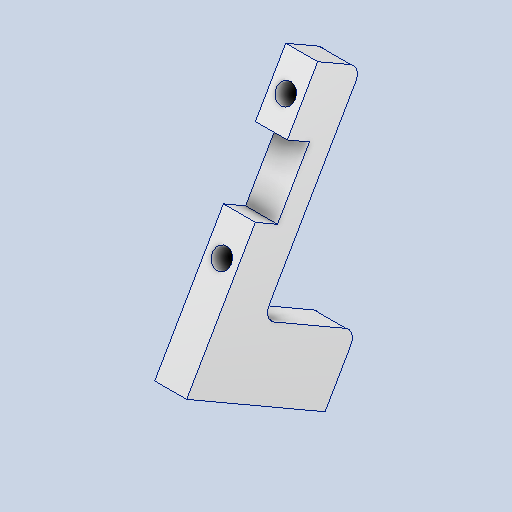
# Autodesk Inventor part: belt_liner_v2_Plate_5
Saved by Autodesk Inventor 2025.2 (Build 292293000, 293)
## iProperties
Created: 2025-01-06
Part Number: belt_liner_v2_Plate_5
Material: アルミニウム 6061
Document SubType Name: Modeling
Designer: haruy
Density: 2.7 g/cm^3
Appearance: アルミニウム - フラット
Author: haruy
Autodesk Inventor part; units mm, degrees
ref_plane "YZ Plane" through (0, 0, 0) normal (1, 0, 0) x (0, 1, 0)
ref_plane "XZ Plane" through (0, 0, 0) normal (0, 1, 0) x (-1, 0, 0)
ref_plane "XY Plane" through (0, 0, 0) normal (0, 0, 1) x (1, 0, 0)
derived "belt_liner_v2_Sketch_Base.ipt"
sketch "スケッチ1" plane through (300, 0, 0) normal (1, 0, 0) x (0, 1, 0)
  circle A0 centre (0, 0) radius 22.36
  circle A1 centre (742.4003, -428.625) radius 23.875 construction
  line L0 (0, 0) -> (0, -985.832)
  line L1 (4.6934, 56.2493) -> (12.1934, 69.2396)
  line L2 (12.1934, 69.2396) -> (479.8471, -200.7604)
  line L3 (479.8471, -200.7604) -> (472.3471, -213.7507)
  line L4 (472.3471, -213.7507) -> (4.6934, 56.2493)
  line L5 (0, 0) -> (742.4003, -428.625)
  line L6 (-43.5991, -27.3958) -> (-51.0991, -40.3862)
  line L7 (-51.0991, -40.3862) -> (711.0033, -480.3862)
  line L8 (711.0033, -480.3862) -> (718.5033, -467.3958)
  line L9 (718.5033, -467.3958) -> (-43.5991, -27.3958)
  line L10 (-64.8558, 113.724) -> (-64.8558, 113.724)
  line L11 (4.6934, 56.2493) -> (0.3513, 58.7562)
  line L12 (0.3513, 58.7562) -> (-2.1487, 54.426)
  line L13 (-2.1487, 54.426) -> (2.1934, 51.9191)
  line L14 (2.1934, 51.9191) -> (4.6934, 56.2493)
  line L15 (472.3471, -213.7507) -> (374.1722, -157.0694)
  line L16 (0, -985.832) -> (0, 0)
  circle A2 centre (0, 0) radius 12.5
  circle A3 centre (0, 0) radius 15
  line L17 (0, 0) -> (0, 0)
  circle A4 centre (0, 0) radius 24.06 construction
  line L18 (0, 0) -> (0, 0)
  line L19 (0, 0) -> (0, 0)
  line L20 (-43.5991, -27.3958) -> (-41.0991, -23.0657)
  line L21 (-41.0991, -23.0657) -> (28.9181, -63.4901)
  line L22 (32.4803, -71.3202) -> (-43.5991, -27.3958)
  line L23 (85.8056, 26.7396) -> (479.8471, -200.7604)
  line L24 (479.8471, -200.7604) -> (482.5971, -195.9972)
  circle A5 centre (742.4003, -428.625) radius 5
  line L25 (718.5033, -467.3958) -> (692.5225, -452.3958)
  line L26 (692.5225, -452.3958) -> (695.0225, -448.0657)
  line L27 (695.0225, -448.0657) -> (721.0033, -463.0657)
  line L28 (721.0033, -463.0657) -> (718.5033, -467.3958)
  circle A6 centre (738.0702, -426.125) radius 5.1
  line L29 (742.4003, -428.625) -> (511.0389, -295.0485)
  circle A7 centre (759.7208, -438.625) radius 5.1
  line L30 (740.6202, -421.7083) -> (762.2708, -434.2083)
  line L31 (735.5202, -430.5417) -> (757.1708, -443.0417)
  circle A8 centre (742.4003, -428.625) radius 22.175 construction
  line L32 (792.3761, -398.5196) -> (776.3761, -426.2324)
  line L33 (776.3761, -426.2324) -> (785.0364, -431.2324)
  line L34 (785.0364, -431.2324) -> (801.0364, -403.5196)
  line L35 (801.0364, -403.5196) -> (792.3761, -398.5196)
  circle A9 centre (738.0702, -426.125) radius 10.1 construction
  circle A10 centre (759.7208, -438.625) radius 10.1 construction
  line L36 (743.1202, -417.3781) -> (764.7708, -429.8781) construction
  line L37 (733.0202, -434.8719) -> (754.6708, -447.3719) construction
  line L38 (743.1202, -417.3781) -> (732.6663, -411.3426) construction
  line L39 (729.3233, -421.075) -> (734.3733, -412.3281) construction
  line L40 (764.7708, -429.8781) -> (773.0938, -434.6834) construction
  line L41 (773.0938, -434.6834) -> (773.431, -434.8781)
  line L42 (0.3513, 58.7562) -> (-2.1487, 54.426)
  line L43 (-2.1487, 54.426) -> (100.4873, -4.8309)
  line L44 (100.4873, -4.8309) -> (102.9873, -0.5007)
  line L45 (102.9873, -0.5007) -> (0.3513, 58.7562)
  line L46 (-51.0991, -40.3862) -> (-51.0991, -619.9209)
  line L47 (754.6708, -447.3719) -> (764.7708, -429.8781)
  line L48 (764.7708, -429.8781) -> (773.431, -434.8781)
  line L49 (773.431, -434.8781) -> (763.331, -452.3719)
  line L50 (763.331, -452.3719) -> (754.6708, -447.3719) construction
  line L51 (479.8471, -200.7604) -> (472.3471, -213.7507)
  line L52 (472.3471, -213.7507) -> (896.6996, -458.7507)
  line L53 (896.6996, -458.7507) -> (904.1996, -445.7603)
  line L54 (904.1996, -445.7603) -> (479.8471, -200.7604)
  line L55 (-12.1522, -2.9282) -> (-38.1087, -47.8862)
  line L56 (-12.1522, -2.9282) -> (25.1838, 61.7396)
  circle A11 centre (38.0844, 34.0842) radius 1.5
  circle A12 centre (59.7351, 21.5842) radius 1.5
  circle A13 centre (711.093, -460.2307) radius 1.5
  circle A14 centre (0, 0) radius 60
  line L57 (54.6948, -84.1458) -> (57.1948, -79.8157)
  line L58 (100.4873, -4.8309) -> (57.1948, -79.8157)
  circle A15 centre (81.3857, 9.0842) radius 1.5
  circle A16 centre (742.4003, -428.625) radius 6 construction
  circle A17 centre (0, 0) radius 24.06 construction
  circle A18 centre (0, 0) radius 24.06
  circle A19 centre (742.4003, -428.625) radius 24.06
  line L59 (754.4303, -407.7884) -> (12.03, 20.8366)
  circle A20 centre (725.8592, -419.075) radius 4
  circle A21 centre (725.8592, -419.075) radius 1.5
  circle A22 centre (742.4003, -428.625) radius 18.525 construction
  circle A23 centre (748.9869, -417.4167) radius 4
  line L60 (737.4369, -437.4219) -> (742.4869, -428.675)
  circle A24 centre (748.9869, -417.4167) radius 1.5
  line L61 (734.3733, -412.3281) -> (737.8233, -406.3526) construction
  line L62 (737.8233, -406.3526) -> (776.881, -428.9026)
  line L63 (773.431, -434.8781) -> (776.881, -428.9026)
  line L64 (737.8233, -406.3526) -> (723.6503, -415.7402)
  line L65 (720.8233, -435.7974) -> (759.881, -458.3474)
  line L66 (720.8233, -435.7974) -> (721.8667, -418.8295)
  line L67 (763.331, -452.3719) -> (759.881, -458.3474)
  circle A25 centre (735.9869, -439.9333) radius 4
  circle A26 centre (735.9869, -439.9333) radius 1.5
  circle A27 centre (300.5299, 58.6531) radius 120
  line L68 (24.7883, 15.78) -> (16.128, 20.78) construction
  line L69 (896.6996, -458.7507) -> (870.7188, -443.7507)
  line L70 (870.7188, -443.7507) -> (868.2188, -448.0808)
  line L71 (868.2188, -448.0808) -> (894.1996, -463.0808)
  line L72 (894.1996, -463.0808) -> (896.6996, -458.7507)
  circle A28 centre (886.7893, -455.9158) radius 1.5
  line L73 (100.4873, -4.8309) -> (102.9873, -0.5007)
  line L74 (102.9873, -0.5007) -> (112.9466, -6.2507)
  line L75 (112.9466, -6.2507) -> (110.4466, -10.5809)
  line L76 (110.4466, -10.5809) -> (100.4873, -4.8309)
  circle A29 centre (878.129, -450.9158) radius 1.5
  circle A30 centre (702.4328, -455.2307) radius 1.5
  line L77 (28.9181, -63.4901) -> (57.1948, -79.8157)
  line L78 (479.8471, -200.7604) -> (482.5971, -195.9972)
  line L79 (121.4466, 8.4717) -> (179.9033, -25.2783)
  line L80 (179.9033, -25.2783) -> (182.4033, -20.9482)
  line L81 (182.4033, -20.9482) -> (123.9466, 12.8018)
  line L82 (123.9466, 12.8018) -> (121.4466, 8.4717)
  circle A31 centre (135.9059, 10.5159) radius 4
  circle A32 centre (135.9059, 10.5159) radius 11
  circle A33 centre (161.8867, -4.4841) radius 4
  circle A34 centre (161.8867, -4.4841) radius 11
  line L83 (131.87, -4.4745) -> (128.37, -10.5366)
  line L84 (128.37, -10.5366) -> (147.4226, -21.5366)
  line L85 (147.4226, -21.5366) -> (150.9226, -15.4745)
  line L86 (150.9226, -15.4745) -> (131.87, -4.4745)
  line L87 (141.3963, -9.9745) -> (137.8963, -16.0366)
  line L88 (157.8508, -19.4745) -> (154.3508, -25.5366)
  line L89 (154.3508, -25.5366) -> (173.4033, -36.5366)
  line L90 (173.4033, -36.5366) -> (176.9033, -30.4745)
  line L91 (176.9033, -30.4745) -> (157.8508, -19.4745)
  line L92 (167.377, -24.9745) -> (163.877, -31.0366)
  line L93 (8.4434, 62.7444) -> (900.4496, -452.2555)
  line L94 (170.4033, -41.7328) -> (167.9033, -46.0629)
  line L95 (111.9466, -7.9828) -> (170.4033, -41.7328)
  line L96 (167.9033, -46.0629) -> (109.4466, -12.3129)
  line L97 (109.4466, -12.3129) -> (111.9466, -7.9828)
  circle A35 centre (117.4059, -21.527) radius 11
  circle A36 centre (117.4059, -21.527) radius 4
  circle A37 centre (143.3867, -36.527) radius 11
  circle A38 centre (143.3867, -36.527) radius 4
  line L98 (140.9322, -2.7783) -> (147.8604, -6.7783)
  line L99 (147.8604, -6.7783) -> (138.3604, -23.2328)
  line L100 (138.3604, -23.2328) -> (131.4322, -19.2328)
  line L101 (131.4322, -19.2328) -> (140.9322, -2.7783)
  line L102 (166.9129, -17.7783) -> (173.8411, -21.7783)
  line L103 (173.8411, -21.7783) -> (164.3411, -38.2328)
  line L104 (164.3411, -38.2328) -> (157.4129, -34.2328)
  line L105 (157.4129, -34.2328) -> (166.9129, -17.7783)
  line L106 (109.4466, -12.3129) -> (96.9466, -33.9636)
  line L107 (96.9466, -33.9636) -> (105.6069, -38.9636)
  line L108 (105.6069, -38.9636) -> (118.1069, -17.3129)
  line L109 (118.1069, -17.3129) -> (109.4466, -12.3129)
  line L110 (109.4466, -12.3129) -> (144.9536, -32.8129)
  line L111 (144.9536, -32.8129) -> (140.9536, -39.7411)
  line L112 (140.9536, -39.7411) -> (105.4466, -19.2411)
  line L113 (105.4466, -19.2411) -> (109.4466, -12.3129)
  line L114 (128.9322, -23.5629) -> (135.8604, -27.5629)
  line L115 (135.8604, -27.5629) -> (134.3604, -30.161)
  line L116 (134.3604, -30.161) -> (127.4322, -26.161)
  line L117 (127.4322, -26.161) -> (128.9322, -23.5629)
  circle A39 centre (-7.7081, -45.2307) radius 1.25
  circle A40 centre (13.9426, -57.7307) radius 1.25
  circle A41 centre (35.5932, -70.2307) radius 1.25
  circle A42 centre (300.5299, 58.6531) radius 130
  line L118 (300.5299, 58.6531) -> (196.6069, 118.6531)
  line L119 (300.5299, 58.6531) -> (184.6188, 27.5948)
  line L120 (300.5299, 58.6531) -> (269.4716, 174.5642)
  line L121 (272.4716, 179.7603) -> (181.6188, 22.3986)
  line L122 (181.6188, 22.3986) -> (176.4227, 25.3986)
  line L123 (176.4227, 25.3986) -> (267.2755, 182.7603)
  line L124 (267.2755, 182.7603) -> (272.4716, 179.7603)
  line L125 (300.5299, 58.6531) -> (235.5299, -53.9302)
  line L126 (791.3761, -400.2516) -> (788.8761, -404.5817)
  line L127 (788.8761, -404.5817) -> (847.3329, -438.3317)
  line L128 (847.3329, -438.3317) -> (849.8329, -434.0016)
  line L129 (849.8329, -434.0016) -> (791.3761, -400.2516)
  line L130 (849.8329, -434.0016) -> (847.3329, -438.3317)
  line L131 (847.3329, -438.3317) -> (867.2188, -449.8129)
  line L132 (867.2188, -449.8129) -> (869.7188, -445.4828)
  line L133 (869.7188, -445.4828) -> (849.8329, -434.0016)
  line L134 (737.8233, -406.3526) -> (868.2188, -448.0808)
  circle A43 centre (742.4003, -428.625) radius 34.06
  line L135 (859.2446, -445.209) -> (862.7446, -439.1468)
  circle A44 centre (742.4869, -428.675) radius 8.5
  line L136 (126.0662, -26.527) -> (134.7264, -31.527)
  line L137 (134.7264, -31.527) -> (137.2264, -27.1969)
  line L138 (137.2264, -27.1969) -> (128.5662, -22.1969)
  line L139 (128.5662, -22.1969) -> (126.0662, -26.527)
  line L140 (253.2022, 236.6791) -> (109.4466, -12.3129)
  line L141 (249.3989, -49.9085) -> (244.3828, -58.5967)
  line L142 (244.3828, -58.5967) -> (167.9033, -46.0629)
  line L143 (181.6188, 22.3986) -> (198.8709, -5.1077)
  line L144 (267.2755, 182.7603) -> (268.3404, 184.6048)
  circle A45 centre (127.0267, 8.1368) radius 1.5
  circle A46 centre (176.8232, -20.6132) radius 1.5
  circle A47 centre (115.0267, -12.6479) radius 1.5
  circle A48 centre (164.8232, -41.3979) radius 1.5
  line L145 (176.4227, 25.3986) -> (179.4227, 30.5948)
  line L146 (179.4227, 30.5948) -> (175.0925, 33.0948)
  line L147 (175.0925, 33.0948) -> (172.0925, 27.8986)
  line L148 (172.0925, 27.8986) -> (176.4227, 25.3986)
  line L149 (267.2755, 182.7603) -> (264.2755, 177.5642)
  line L150 (264.2755, 177.5642) -> (259.9453, 180.0642)
  line L151 (259.9453, 180.0642) -> (262.9453, 185.2603)
  line L152 (262.9453, 185.2603) -> (267.2755, 182.7603)
  circle A49 centre (263.6104, 181.4122) radius 1.5
  line L153 (268.3404, 184.6048) -> (262.9453, 185.2603)
  line L154 (262.9453, 185.2603) -> (242.1446, 174.8045)
  circle A50 centre (175.7576, 29.2467) radius 1.5
  line L155 (894.1996, -463.0808) -> (718.5033, -467.3958)
  line L156 (695.0225, -448.0657) -> (722.8562, -416.4327)
  line L157 (870.7188, -443.7507) -> (868.2188, -448.0808)
  line L158 (868.2188, -448.0808) -> (861.2906, -444.0808)
  line L159 (861.2906, -444.0808) -> (863.7906, -439.7507)
  line L160 (863.7906, -439.7507) -> (870.7188, -443.7507)
  line L161 (-33.3539, -27.641) -> (-48.3539, -27.641)
  line L162 (-48.3539, -27.641) -> (-48.3539, -280.141)
  line L163 (-48.3539, -280.141) -> (-33.3539, -280.141)
  line L164 (-33.3539, -280.141) -> (-33.3539, -27.641)
  line L165 (331.6461, -265.141) -> (-48.3539, -265.141)
  line L166 (-48.3539, -265.141) -> (-48.3539, -280.141)
  line L167 (-48.3539, -280.141) -> (331.6461, -280.141)
  line L168 (331.6461, -280.141) -> (331.6461, -265.141)
  line L169 (-20.7882, -57.8862) -> (-13.2882, -44.8958)
  line L170 (5.1926, -72.8862) -> (12.6926, -59.8958)
  line L171 (-48.3539, -74.641) -> (-71.3539, -74.641)
  line L172 (-71.3539, -74.641) -> (-71.3539, -134.641)
  line L173 (-71.3539, -134.641) -> (-48.3539, -134.641)
  line L174 (-48.3539, -134.641) -> (-48.3539, -74.641)
  line L175 (-48.3539, -94.641) -> (-93.3539, -94.641)
  line L176 (-93.3539, -94.641) -> (-93.3539, -114.641)
  line L177 (-93.3539, -114.641) -> (-48.3539, -114.641)
  line L178 (-48.3539, -114.641) -> (-48.3539, -94.641)
  line L179 (-33.3539, -74.641) -> (-48.3539, -74.641)
  line L180 (-93.3539, -104.641) -> (-48.3539, -104.641)
  line L181 (-57.3539, -244.641) -> (-62.3539, -244.641)
  line L182 (-62.3539, -244.641) -> (-62.3539, -254.641)
  line L183 (-62.3539, -254.641) -> (-57.3539, -254.641)
  line L184 (-57.3539, -254.641) -> (-57.3539, -244.641)
  line L185 (-48.3539, -236.1427) -> (-53.3539, -236.1427)
  line L186 (-53.3539, -236.1427) -> (-53.3539, -262.0507)
  line L187 (-53.3539, -262.0507) -> (-48.3539, -262.0507)
  line L188 (-48.3539, -262.0507) -> (-48.3539, -236.1427)
  line L189 (-50.8539, -236.1427) -> (-50.8539, -262.0507)
  line L190 (301.6461, -265.141) -> (301.6461, -280.141)
  line L191 (331.6461, -280.141) -> (364.1684, -280.141)
  line L192 (364.1684, -280.141) -> (371.6684, -267.1506)
  line L193 (331.6461, -265.141) -> (338.1877, -265.141)
  line L194 (338.1877, -265.141) -> (345.6877, -252.1506)
  line L195 (-62.3539, -249.641) -> (-57.3539, -249.641)
  line L196 (-89.3539, 250.2187) -> (-109.3539, 250.2187)
  line L197 (-109.3539, 250.2187) -> (-109.3539, -699.6003)
  line L198 (-109.3539, -699.6003) -> (-89.3539, -699.6003)
  line L199 (-89.3539, -699.6003) -> (-89.3539, 250.2187)
  line L200 (263.6104, 181.4122) -> (-89.3539, 181.4122)
  line L201 (-26.7774, -265.2895) -> (-29.2892, -274.9689)
  line L202 (-29.2892, -274.9689) -> (688.5358, -461.2425)
  line L203 (688.5358, -461.2425) -> (691.0476, -451.5631)
  line L204 (691.0476, -451.5631) -> (-26.7774, -265.2895)
  line L205 (-48.3539, -157.9697) -> (-50.3539, -157.9697)
  line L206 (-50.3539, -157.9697) -> (-50.3539, -198.399)
  line L207 (-50.3539, -198.399) -> (-48.3539, -198.399)
  line L208 (-48.3539, -198.399) -> (-48.3539, -157.9697)
  line L209 (-48.3539, -162.0415) -> (22.7461, -162.0415)
  line L210 (22.7461, -162.0415) -> (22.7461, -204.0415)
  line L211 (22.7461, -204.0415) -> (-48.3539, -204.0415)
  line L212 (-48.3539, -204.0415) -> (-48.3539, -162.0415)
  line L213 (-48.3539, -165.4337) -> (-51.3539, -165.4337)
  line L214 (-51.3539, -165.4337) -> (-51.3539, -191.4337)
  line L215 (-51.3539, -191.4337) -> (-48.3539, -191.4337)
  line L216 (-48.3539, -191.4337) -> (-48.3539, -165.4337)
  line L217 (-51.3539, -177.4949) -> (-75.6539, -177.4949)
  line L218 (-75.6539, -177.4949) -> (-75.6539, -187.4949)
  line L219 (-75.6539, -187.4949) -> (-51.3539, -187.4949)
  line L220 (-51.3539, -187.4949) -> (-51.3539, -177.4949)
  line L221 (-56.3539, -167.251) -> (-66.3539, -167.251)
  line L222 (-66.3539, -167.251) -> (-66.3539, -197.251)
  line L223 (-66.3539, -197.251) -> (-56.3539, -197.251)
  line L224 (-56.3539, -197.251) -> (-56.3539, -167.251)
  line L225 (-66.3539, -156.2112) -> (-72.3539, -156.2112)
  line L226 (-72.3539, -156.2112) -> (-72.3539, -222.3443)
  line L227 (-72.3539, -222.3443) -> (-66.3539, -222.3443)
  line L228 (-66.3539, -222.3443) -> (-66.3539, -156.2112)
  circle A51 centre (986.855, -337.5969) radius 120
  line L229 (54.6948, -84.1458) -> (57.1948, -79.8157)
  line L230 (57.1948, -79.8157) -> (67.1541, -85.5657)
  line L231 (67.1541, -85.5657) -> (64.6541, -89.8958)
  line L232 (64.6541, -89.8958) -> (54.6948, -84.1458)
  line L233 (-43.5991, -27.3958) -> (2.1934, 51.9191)
  line L234 (-19.4528, 14.4267) -> (142.0763, -78.8321)
  circle A52 centre (74.6188, -7.5516) radius 15
  line L235 (64.6541, -89.8958) -> (112.9466, -6.2507)
  circle A53 centre (74.6188, -7.5516) radius 22
  circle A54 centre (67.1497, -35.5733) radius 5
  circle A55 centre (103.6165, -12.411) radius 5
  circle A56 centre (65.324, -78.7356) radius 5
  circle A57 centre (11.7598, -74.0723) radius 15
  circle A58 centre (48.162, -57.4928) radius 15
  circle A59 centre (48.162, -57.4928) radius 22
  circle A60 centre (0, 0) radius 24.06
  line L236 (854.2611, -442.3317) -> (857.7611, -436.2696) construction
  line L237 (861.2906, -444.0808) -> (863.7906, -439.7507)
  line L238 (863.7906, -439.7507) -> (857.7284, -436.2507)
  line L239 (857.7284, -436.2507) -> (855.2284, -440.5808)
  line L240 (855.2284, -440.5808) -> (861.2906, -444.0808)
  point P0 (732.6663, -411.3426)
  point P1 (-0.8987, 56.5911)
  point P2 (114.1069, -24.2411)
  point P3 (136.7264, -28.0629)
  point P4 (128.0662, -23.0629)
  point P5 (-30.6087, -34.8958)
  point P6 (-40.8539, -37.641)
  point P7 (-40.8539, -272.641)
  point P8 (321.6461, -272.641)
  point P9 (311.6461, -272.641)
  point P10 (351.0226, -263.891)
  point P11 (359.6829, -268.891)
  point P12 (-18.3539, -272.641)
  point P13 (680.1123, -453.891)
  dimension "d1" = 1
  measures "d1" distance between parallel lines of L116 L136
extrude "押し出し1" add sketch "スケッチ1" against normal blind 5 contours L106 L112 A35 L108 L59 | L59 L108 L107 L106 | L106 L96 A35 L112 | A35 L112 L108 | A35 L96 L108 A36 L112 | L112 A36 L96 L139 L136 A35 | A35 L136 A37 L112 | L108 A36 L112 | A37 L136 L137 L96 L111 A38 L112 | A36 L108 | A36 L108 | L96 A36 L108 | A38 L111 picked at (109.0217, -22.1019) picked at (141.5428, -35.1993)
sketch "スケッチ2" plane through (300, 114.1069, -24.2411) normal (0, -0.5, -0.8660254) x (-1, 0, 0)
  line L0 (0, -10) -> (5, -10) projected
  line L1 (5, 31) -> (5, 0) projected
  line L2 (0, 0) -> (0, 31) projected
  point P0 (300, -110.94)
  point P1 (2.5, 6)
  point P2 (2.5, 26)
  dimension "d4" = 16
  dimension "d5" = 20
  dimension "d6" = 2.5
  dimension "d7" = 2.5
  measures "d4" distance from line of point (2.5, 6) L0
  measures "d5" distance of point (2.5, 26) point (2.5, 6)
  measures "d6" distance from line of point (2.5, 6) L1
  measures "d7" distance from line of point (2.5, 26) L2
hole "穴1" at (297.5, 119.303, -27.2411) at (297.5, 136.6235, -37.2411) direction (0, 0.5, 0.8660254) diameter 3 end through all
fillet "フィレット1" radius 2 3 edges at (297.5, 105.6069, -38.9636) (297.5, 114.1069, -24.2411) (297.5, 140.9536, -39.7411)
equation "\"d7\" = d6"
